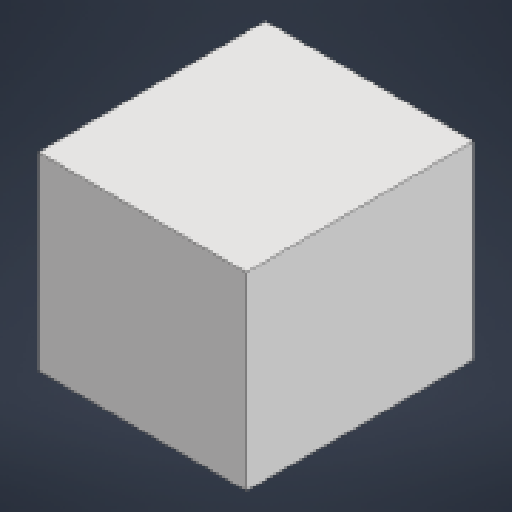
# Autodesk Inventor part: PCB_Housing_05_V4
Saved by Autodesk Inventor 2026.2 (Build 302298000, 298)
## iProperties
Created: 2026-03-17
Part Number: PCB_Housing_05_V4
Material: Generic
Document SubType Name: Modeling
Designer: vckot
Density: 1 g/cm^3
Appearance: Default
Author: vckot
Autodesk Inventor part; units mm, degrees
ref_plane "YZ Plane" through (0, 0, 0) normal (1, 0, 0) x (0, 1, 0)
ref_plane "XZ Plane" through (0, 0, 0) normal (0, 1, 0) x (-1, 0, 0)
ref_plane "XY Plane" through (0, 0, 0) normal (0, 0, 1) x (1, 0, 0)
sketch "Sketch1" plane through (0, 0, 0) normal (0, 1, 0) x (-1, 0, 0)
  line L0 (11, 11.5) -> (-11, 11.5)
  line L1 (-11, 11.5) -> (-11, -11.5)
  line L2 (-11, -11.5) -> (11, -11.5)
  line L3 (11, -11.5) -> (11, 11.5)
  line L4 (11, 11.5) -> (-11, -11.5) construction
  line L5 (-11, 11.5) -> (11, -11.5) construction
  point P0 (0, 0)
  dimension "d0" = 22
  dimension "d1" = 23
  constraints: 12 end point, 2 midpoint, 2 parallel, 1 horizontal, 1 perpendicular
  measures "d0" distance of L2.end L1.end
  measures "d1" distance of L1.end L0.end
extrude "Extrusion1" add sketch "Sketch1" along normal blind 22
body "Solid1"
